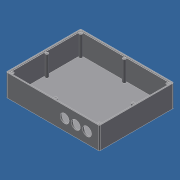
# Autodesk Inventor part: Box
Saved by Autodesk Inventor 2015 SP2 (Build 190223200, 223)
## iProperties
Created: 2017-06-14
Part Number: Box
Project: Nom Projet
Material: .
Description: Nom pièce
Document SubType Name: Modeling
Designer: Francis-Lucien-Hugue
Authority: brut Ø
Density: 0.001 g/cm^3
Appearance: Par défaut
Material number: ---
Author: Francis-Lucien-Hugue
Autodesk Inventor part; units mm, degrees
ref_plane "Plan YZ" through (0, 0, 0) normal (1, 0, 0) x (0, 1, 0)
ref_plane "Plan XZ" through (0, 0, 0) normal (0, 1, 0) x (-1, 0, 0)
ref_plane "Plan XY" through (0, 0, 0) normal (0, 0, 1) x (1, 0, 0)
sketch "Esquisse1" plane through (0, 0, 0) normal (0, 0, 1) x (1, 0, 0)
  line L0 (-125, -100) -> (125, -100)
  line L1 (125, -100) -> (125, 100)
  line L2 (125, 100) -> (-125, 100)
  line L3 (-125, 100) -> (-125, -100)
  line L4 (-125, -100) -> (125, 100) construction
  line L5 (125, -100) -> (-125, 100) construction
  point P0 (0, 0)
  dimension "d0" = 250
  dimension "d1" = 200
  constraints: 12 end point, 2 midpoint, 2 parallel, 1 horizontal, 1 perpendicular
  measures "d0" distance of L2.end L1.end
  measures "d1" distance of L1.end L0.end
extrude "Extrusion1" add sketch "Esquisse1" along normal blind 59
sketch "Esquisse6" plane through (0, 0, 59) normal (0, 0, 1) x (1, 0, 0)
  line L0 (-120.7, -95.7) -> (120.7, -95.7)
  line L1 (120.7, -95.7) -> (120.7, 95.7)
  line L2 (120.7, 95.7) -> (-120.7, 95.7)
  line L3 (-120.7, 95.7) -> (-120.7, -95.7)
  line L4 (-120.7, -95.7) -> (120.7, 95.7) construction
  line L5 (120.7, -95.7) -> (-120.7, 95.7) construction
  line L6 (125, 100) -> (-125, 100) projected
  line L7 (125, -100) -> (125, 100) projected
  point P0 (0, 0)
  dimension "d4" = 4.3
  dimension "d5" = 4.3
  constraints: 12 end point, 2 midpoint, 2 parallel, 1 horizontal, 1 perpendicular
  measures "d4" distance between parallel lines of L6 L2
  measures "d5" distance between parallel lines of L7 L1
extrude "Extrusion2" cut sketch "Esquisse6" against normal blind 57
sketch "Esquisse7" plane through (0, 0, 59) normal (0, 0, 1) x (1, 0, 0)
  line L0 (-121.7, -96.7) -> (121.7, -96.7)
  line L1 (121.7, -96.7) -> (121.7, 96.7)
  line L2 (121.7, 96.7) -> (-121.7, 96.7)
  line L3 (-121.7, 96.7) -> (-121.7, -96.7)
  line L4 (-121.7, -96.7) -> (121.7, 96.7) construction
  line L5 (121.7, -96.7) -> (-121.7, 96.7) construction
  line L6 (125, 100) -> (-125, 100) projected
  line L7 (125, -100) -> (125, 100) projected
  point P0 (0, 0)
  dimension "d8" = 3.3
  dimension "d9" = 3.3
  constraints: 12 end point, 2 midpoint, 2 parallel, 1 horizontal, 1 perpendicular
  measures "d8" distance between parallel lines of L6 L2
  measures "d9" distance between parallel lines of L7 L1
extrude "Extrusion3" cut sketch "Esquisse7" against normal blind 2
fillet "Congé1" radius 3 12 edges at (-120.7, 95.7, 29.5) (-121.7, 96.7, 58) (-125, 100, 29.5) (120.7, 95.7, 29.5) (121.7, 96.7, 58) (120.7, -95.7, 29.5) (121.7, -96.7, 58) (-121.7, -96.7, 58) (-120.7, -95.7, 29.5) (-125, -100, 29.5) (125, -100, 29.5) (125, 100, 29.5)
sketch "Esquisse9" plane through (0, 0, 2) normal (0, 0, 1) x (1, 0, 0)
  line L0 (118.7, -96.7) -> (-118.7, -96.7) projected
  line L1 (-121.7, -93.7) -> (-121.7, 93.7) projected
  circle A0 centre (-116.7, -91.7) radius 4
  line L2 (0, 0) -> (0, 94.7693)
  line L3 (0, 0) -> (-121.7, 0)
  circle A1 centre (-116.7, 91.7) radius 4
  circle A2 centre (116.7, -91.7) radius 4
  circle A3 centre (116.7, 91.7) radius 4
  dimension "d15" = 5
  dimension "d16" = 5
  dimension "d17" = 8
  constraints: 6 symmetric about line, 4 centre point, 4 coincident, 4 end point, 1 midpoint, 1 vertical, 3 other
  measures "d15" distance from line of L0 point (-116.7, -91.7)
  measures "d16" distance from line of L1 point (-116.7, -91.7)
  measures "d17" diameter of A0
extrude "Extrusion4" add sketch "Esquisse9" along normal blind 55
sketch "Esquisse10" plane through (0, 0, 2) normal (0, 0, 1) x (1, 0, 0)
  line L0 (118.7, -96.7) -> (-118.7, -96.7) projected
  line L1 (121.7, 93.7) -> (121.7, -93.7) projected
  line L2 (-121.7, -93.7) -> (-121.7, 93.7) projected
  circle A0 centre (0, -91.7) radius 4
  line L3 (0, 0) -> (121.7, 0)
  circle A1 centre (0, 91.7) radius 4
  dimension "d20" = 5
  dimension "d21" = 243.4
  dimension "d22" = 121.7
  dimension "d23" = 8
  constraints: 2 centre point, 2 coincident, 2 end point, 2 symmetric about line, 1 midpoint, 1 other
  measures "d20" distance from line of L0 point (0, -91.7)
  measures "d21" distance between parallel lines of L1 L2
  measures "d22" distance from line of L2 point (0, -91.7)
  measures "d23" diameter of A0
extrude "Extrusion5" add sketch "Esquisse10" along normal blind 55
sketch "Esquisse14" plane through (0, 0, 2) normal (0, 0, 1) x (1, 0, 0)
  line L0 (-120.7, 91.7) -> (-120.7, -91.7) projected
  line L1 (-116.7, -95.7) -> (0, -95.7) projected
  line L2 (0, 95.7) -> (-116.7, 95.7) projected
  circle A0 centre (-115.7, 0) radius 4
  circle A1 centre (0, 91.7) radius 4 projected
  line L3 (0, 0) -> (0, 91.7)
  circle A2 centre (115.7, 0) radius 4
  dimension "d45" = 5
  dimension "d46" = 191.4
  dimension "d47" = 95.7
  dimension "d48" = 8
  constraints: 2 centre point, 2 coincident, 2 end point, 2 symmetric about line, 1 vertical, 1 vertical alignment, 1 other
  measures "d45" distance from line of L0 point (-115.7, 0)
  measures "d46" distance between parallel lines of L1 L2
  measures "d47" distance from line of L1 point (-115.7, 0)
  measures "d48" diameter of A0
extrude "Extrusion7" add sketch "Esquisse14" along normal blind 55 contours A0 | A2
sketch "Esquisse12" plane through (0, 91.7, 57) normal (0, 0, 1) x (1, 0, 0)
  circle A0 centre (0, 0) radius 4 projected
  arc A1 (116.7, 4) -> (120.7, 0) centre (116.7, 0) ccw projected
  arc A2 (120.7, -183.4) -> (116.7, -187.4) centre (116.7, -183.4) ccw projected
  arc A3 (-120.7, 0) -> (-116.7, 4) centre (-116.7, 0) ccw projected
  circle A4 centre (0, -183.4) radius 4 projected
  arc A5 (-116.7, -187.4) -> (-120.7, -183.4) centre (-116.7, -183.4) ccw projected
  circle A6 centre (-115.7, -91.7) radius 4 projected
  circle A7 centre (115.7, -91.7) radius 4 projected
  point P0 (0, -91.7)
  point P1 (0, 4)
  point P2 (0, -187.4)
  constraints: 8 coincident, 2 vertical alignment
hole "Perçage1" at (0, 91.7, 57) at (116.7, 91.7, 57) at (116.7, -91.7, 57) at (-116.7, 91.7, 57) at (0, -91.7, 57) at (-116.7, -91.7, 57) at (115.7, 0, 57) at (-115.7, 0, 57) direction (0, 0, -1) diameter 2.459 depth 20 tip angle 118 thread size "M3x0.5" class "6H" standard "ISO M"
sketch "Esquisse13" plane through (-122, -100, 0) normal (0, -1, 0) x (1, 0, 0)
  line L0 (244, 59) -> (244, 0) projected
  line L1 (0, 59) -> (244, 59) projected
  line L2 (0, 0) -> (244, 0) projected
  circle A0 centre (154, 29.5) radius 12
  circle A1 centre (184, 29.5) radius 12
  circle A2 centre (214, 29.5) radius 12
  point P0 (122, 0)
  dimension "d33" = 30
  dimension "d34" = 30
  dimension "d35" = 30
  dimension "d36" = 59
  dimension "d37" = 29.5
  dimension "d38" = 29.5
  dimension "d39" = 29.5
  dimension "d40" = 24
  dimension "d41" = 24
  dimension "d42" = 24
  constraints: 3 centre point, 3 coincident
  measures "d33" distance from line of L0 point (214, 29.5)
  measures "d34" distance of point (184, 29.5) point (214, 29.5)
  measures "d35" distance of point (154, 29.5) point (184, 29.5)
  measures "d36" distance between parallel lines of L1 L2
  measures "d37" distance from line of L2 point (154, 29.5)
  measures "d38" distance from line of L2 point (184, 29.5)
  measures "d39" distance from line of L2 point (214, 29.5)
  measures "d40" diameter of A0
  measures "d41" diameter of A1
  measures "d42" diameter of A2
extrude "Extrusion6" cut sketch "Esquisse13" against normal blind 10
